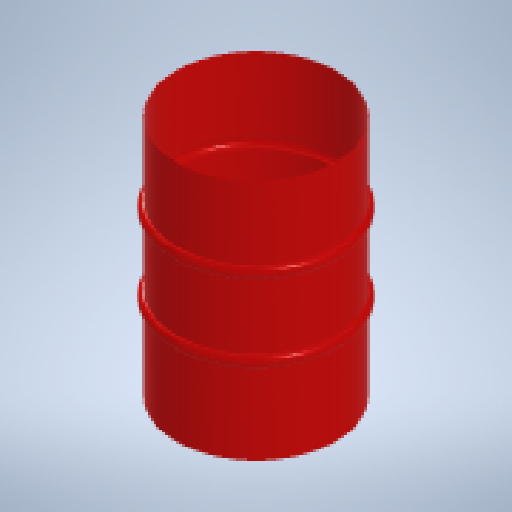
# Autodesk Inventor part: Fass
Saved by Autodesk Inventor 2024 (Build 280153000, 153)
## iProperties
Created: 2023-11-30
Part Number: Fass
Material: Generic
Document SubType Name: Modeling
Designer: Daniel Nussbaum
Density: 1 g/cm^3
Appearance: Default
Author: Daniel Nussbaum
Autodesk Inventor part; units mm, degrees
ref_plane "YZ Plane" through (0, 0, 0) normal (1, 0, 0) x (0, 1, 0)
ref_plane "XZ Plane" through (0, 0, 0) normal (0, 1, 0) x (-1, 0, 0)
ref_plane "XY Plane" through (0, 0, 0) normal (0, 0, 1) x (1, 0, 0)
sketch "Sketch1" plane through (0, 0, 0) normal (0, 0, 1) x (1, 0, 0)
  line L0 (0, 0) -> (0, 15)
  line L1 (0, 850) -> (-280, 850)
  line L2 (-280, 850) -> (-280, 595)
  line L3 (-280, 0) -> (0, 0)
  arc A0 (-280, 324) -> (-280, 284) centre (-274.1667, 304) ccw
  line L4 (-280, 0) -> (-278, 0)
  line L5 (-278, 0) -> (-278, 15)
  line L6 (-278, 15) -> (0, 15)
  arc A1 (-280, 595) -> (-280, 555) centre (-274.1667, 575) ccw
  line L7 (-278, 15) -> (-280, 15)
  line L8 (-280, 15) -> (-280, 0)
  line L9 (0, 15) -> (0, 850)
  line L10 (-279, 15) -> (-279, 284.96)
  line L11 (-279, 849) -> (-1, 849)
  line L12 (-1, 849) -> (-1, 15)
  line L13 (-279, 849) -> (-279, 850)
  line L14 (-279, 16) -> (-1, 16)
  line L15 (-1, 16) -> (0, 16)
  arc A2 (-279.72, 594.04) -> (-279.72, 555.96) centre (-274.1667, 575) ccw
  line L16 (-279.72, 555.96) -> (-279, 555.96)
  line L17 (-279.72, 594.04) -> (-279, 594.04)
  line L18 (-279, 594.04) -> (-279, 849)
  line L19 (-279, 555.96) -> (-279, 594.04)
  line L20 (-280, 556.0439) -> (-280, 555)
  line L21 (-280, 593.9561) -> (-280, 556.0439)
  line L22 (-280, 595) -> (-280, 593.9561)
  line L23 (-280, 555) -> (-280, 324)
  arc A3 (-279.72, 323.04) -> (-280, 285.0439) centre (-274.1667, 304) ccw
  line L24 (-279.72, 323.04) -> (-279, 323.04)
  line L25 (-279.72, 284.96) -> (-279, 284.96)
  arc A4 (-280, 285.0439) -> (-279.72, 284.96) centre (-274.1667, 304) ccw
  line L26 (-280, 284) -> (-280, 15)
  line L27 (-279, 284.96) -> (-279, 555.96)
  line L28 (-280, 322.9561) -> (-280, 284)
  line L29 (-280, 324) -> (-280, 322.9561)
  point P0 (-295, 304)
  point P1 (-295, 575)
  dimension "d0" = 850
  dimension "d1" = 280
  dimension "d2" = 40
  dimension "d3" = 15
  dimension "d5" = 2
  dimension "d6" = 15
  dimension "d7" = 284
  dimension "d8" = 40
  dimension "d9" = 15
  dimension "d10" = 255
  dimension "d14" = 1
  dimension "d15" = 1
  dimension "d16" = 1
  dimension "d17" = 1
  constraints: 60 end point, 49 perpendicular, 15 point on circle, 14 point on line, 5 centre point, 2 vertical, 1 horizontal, 1 other
  measures "d0" distance of L0.start L1.start
  measures "d1" distance of L1.start L1.end
  measures "d2" distance of L23.end L26.start
  measures "d3" distance from line of L2 point (-295, 304)
  measures "d5" distance of L3.start L4.end
  measures "d6" distance of L4.end L5.end
  measures "d7" distance from line of L26.start L3
  measures "d8" distance of L2.end L20.end
  measures "d9" distance from line of L2 point (-295, 575)
  measures "d10" distance from line of L1 L2.end
  measures "d14" distance between parallel lines of L2 L10
  measures "d15" distance between parallel lines of L6 L14
  measures "d16" radial gap between concentric circles of A1 A2
  measures "d17" radial gap between concentric circles of A0 A3
revolve "Revolution1" add sketch "Sketch1" angle 360 about axis through (0, 15, 0) along (0, 1, 0) contours L6 L12 L15 L9 | L3 L8 L7 L5 | L6 L7 L10 L14 L12 | L26 L28 A4 L25 L10 L7 | L13 L18 L17 A2 L22 L2 L1 | A0 L29 A3 L28 | L23 L20 A2 L16 L27 L24 A3 L29 | L22 A2 L20 A1
ref_plane "Work Plane2" through (0, 200, 0) normal (0, -1, 0) x (1, 0, 0)
sketch "Sketch5" plane through (0, 200, 0) normal (0, -1, 0) x (1, 0, 0)
  circle A0 centre (0, 0) radius 280 projected
  circle A1 centre (0, 0) radius 280 projected
  circle A2 centre (0, 0) radius 280 projected
  circle A3 centre (0, 0) radius 280 projected
  circle A4 centre (0, 0) radius 290
  line L0 (0, 0) -> (-276.1822, 39.5525)
  line L1 (0, 0) -> (276.1822, 39.5525)
  line L2 (0, 0) -> (0, 290)
  circle A5 centre (0, 0) radius 279 projected
  line L3 (-276.1822, 39.5525) -> (-287.0711, 41.1119)
  line L4 (276.1822, 39.5525) -> (287.0711, 41.1119)
  circle A6 centre (0, 0) radius 390
  line L5 (-287.0711, 41.1119) -> (-386.0611, 55.2884)
  line L6 (276.1822, 39.5525) -> (386.0611, 55.2884)
  dimension "d29" = 10
  dimension "d30" = 81.85
  dimension "d31" = 163.7
  dimension "d32" = 100
  constraints: 14 end point, 7 point on circle, 2 centre point, 1 point on line, 1 vertical
  measures "d29" radial gap between concentric circles of A0 A4
  measures "d30" angle of L1 L2
  measures "d31" angle of L0 L1
  measures "d32" radial gap between concentric circles of A4 A6
extrude "Extrusion2" cut sketch "Sketch5" against normal blind 480 contours L4 A5 L2 A0 | A0 L2 A4 L4 | L3 A4 L2 A0 | A0 L2 A5 L3 | A4 L5 A6 L6 picked at (240.4346, 263.1578)
body "Solid1"
